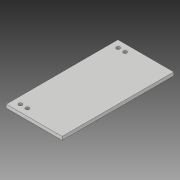
# Autodesk Inventor part: shelf
Saved by Autodesk Inventor 2019 (Build 230136000, 136)
## iProperties
Created: 2019-05-07
Part Number: shelf
Material: Generic
Document SubType Name: Modeling
Designer: devon
Density: 1 g/cm^3
Appearance: Default
Author: devon
Autodesk Inventor part; units mm, degrees
ref_plane "YZ Plane" through (0, 0, 0) normal (1, 0, 0) x (0, 1, 0)
ref_plane "XZ Plane" through (0, 0, 0) normal (0, 1, 0) x (-1, 0, 0)
ref_plane "XY Plane" through (0, 0, 0) normal (0, 0, 1) x (1, 0, 0)
sketch "Sketch1" plane through (0, 0, 0) normal (0, 1, 0) x (-1, 0, 0)
  line L0 (-50, 100) -> (50, 100)
  line L1 (50, 100) -> (50, -100)
  line L2 (50, -100) -> (-50, -100)
  line L3 (-50, -100) -> (-50, 100)
  line L4 (-50, 100) -> (50, -100) construction
  line L5 (50, 100) -> (-50, -100) construction
  point P0 (0, 0)
  dimension "d0" = 200
  dimension "d1" = 100
  constraints: 12 end point, 2 midpoint, 2 parallel, 1 horizontal, 1 perpendicular
  measures "d0" distance of L0.end L1.end
  measures "d1" distance of L0.start L0.end
extrude "Extrusion1" add sketch "Sketch1" along normal blind 6
sketch "Sketch2" plane through (0, 6, 0) normal (0, 1, 0) x (1, 0, 0)
  circle A0 centre (-37, -87.5) radius 3.25
  circle A1 centre (-24.5, -87.5) radius 3.25
  circle A2 centre (-37, 87.5) radius 3.25
  circle A3 centre (-24.5, 87.5) radius 3.25
  line L0 (-50, 100) -> (-50, -100) projected
  line L1 (-50, -100) -> (50, -100) projected
  line L2 (50, 100) -> (-50, 100) projected
  point P0 (0, 0)
  dimension "d4" = 6.5
  dimension "d5" = 6.5
  dimension "d6" = 12.5
  dimension "d7" = 13
  dimension "d8" = 12.5
  dimension "d9" = 12.5
  dimension "d10" = 6.5
  dimension "d11" = 6.5
  dimension "d12" = 12.5
  dimension "d13" = 13
  dimension "d14" = 12.5
  dimension "d15" = 12.5
  constraints: 4 centre point
  measures "d4" diameter of A0
  measures "d5" diameter of A1
  measures "d6" distance of A1.centre A0.centre
  measures "d7" distance from line of L0 A0.centre
  measures "d8" distance from line of L1 A0.centre
  measures "d9" distance from line of L1 A1.centre
  measures "d10" diameter of A2
  measures "d11" diameter of A3
  measures "d12" distance of A3.centre A2.centre
  measures "d13" distance from line of L0 A2.centre
  measures "d14" distance from line of L2 A2.centre
  measures "d15" distance from line of L2 A3.centre
extrude "Extrusion2" cut sketch "Sketch2" against normal through all
body "Solid1"
